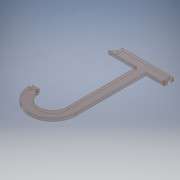
# Autodesk Inventor part: Liu_Inital_J
Saved by Autodesk Inventor 2017 (Build 210142000, 142)
## iProperties
Created: 2016-09-21
Part Number: Liu_Inital_J
Material: Polycarbonate, Smoke
Document SubType Name: Modeling
Designer: jliu
Density: 1.2 g/cm^3
Appearance: Polycarbonate - Smoked
Mass: 7.34155 g
Surface Area: 52.246 cm^2
Volume: 6.11796 cm^3
Author: jliu
Autodesk Inventor part; units mm, degrees
ref_plane "YZ Plane" through (0, 0, 0) normal (1, 0, 0) x (0, 1, 0)
ref_plane "XZ Plane" through (0, 0, 0) normal (0, 1, 0) x (-1, 0, 0)
ref_plane "XY Plane" through (0, 0, 0) normal (0, 0, 1) x (1, 0, 0)
sketch "Sketch1" plane through (0, 0, 0) normal (0, 0, 1) x (1, 0, 0)
  line L0 (5, 37.5) -> (5, -36.707)
  line L1 (-0.001, -37.5) -> (-0.001, 47.5) construction
  line L2 (-5.0021, 37.5) -> (-5.0021, -36.707)
  arc A0 (-44.9937, -37.5) -> (5, -36.707) centre (-19.9969, -37.1035) ccw
  arc A1 (-34.9916, -37.5) -> (-5.0021, -36.707) centre (-19.9969, -37.1035) ccw
  line L3 (5, 37.5) -> (24.9895, 37.5)
  line L4 (-24.9916, 47.5) -> (24.9895, 47.5)
  line L5 (-41.9937, -37.5) -> (-43.4937, -34.9019)
  line L6 (-41.9937, -37.5) -> (-38.9937, -37.5) construction
  line L7 (-44.9937, -37.5) -> (-41.9937, -37.5)
  line L8 (-34.9916, -37.5) -> (-37.9916, -37.5)
  line L9 (-37.9916, -37.5) -> (-36.4916, -34.9019)
  line L10 (-37.9916, -37.5) -> (-34.9916, -37.5) construction
  line L11 (-43.4937, -34.9019) -> (-36.4916, -34.9019)
  line L12 (-34.9916, -37.5) -> (-34.9916, 37.5) construction
  line L13 (-34.9916, -37.5) -> (40.0084, -37.5) construction
  line L14 (-5.0021, 37.5) -> (5, 37.5) construction
  line L15 (-34.9916, 37.5) -> (-5.0021, 37.5)
  line L16 (-34.9916, 37.5) -> (-20.8495, 37.5) construction
  line L17 (-29.9916, 42.5) -> (-29.9916, 47.5)
  line L18 (-29.9916, 47.5) -> (-24.9916, 47.5)
  line L19 (-34.9916, 37.5) -> (-29.9916, 42.5)
  line L20 (24.9895, 44.5) -> (21.9895, 46.2321)
  line L21 (24.9895, 40.5) -> (21.9895, 38.7679)
  line L22 (21.9895, 46.2321) -> (21.9895, 38.7679)
  line L23 (24.9895, 44.5) -> (24.9895, 47.5)
  line L24 (24.9895, 40.5) -> (24.9895, 37.5)
  point P0 (0, 0)
  dimension "d5" = 5
  dimension "d7" = 50
  dimension "d8" = 25
  dimension "d9" = 15
  dimension "d10" = 15
  dimension "d16" = 37.5
  dimension "d17" = 10
  dimension "d18" = 75
  dimension "d20" = 3
  dimension "d22" = 3
  dimension "d25" = 60
  dimension "d26" = 60
  dimension "d28" = 75
  dimension "d29" = 90
  dimension "d31" = 10
  dimension "d32" = 45
  dimension "d33" = 5
  dimension "d39" = 3
  dimension "d41" = 3
  dimension "d42" = 60
  dimension "d43" = 60
  dimension "d45" = 3
  dimension "d46" = 19.9895
  dimension "d47" = 24.9906
  dimension "d48" = 45.839
  constraints: 50 end point, 9 horizontal, 5 equal length, 4 point on circle, 3 collinear, 3 parallel, 3 symmetric about line, 3 vertical, 2 centre point, 1 coincident, 1 point on line
  measures "d5" distance from line of L0 point (0, 0)
  measures "d7" distance of L0.end L7.start
  measures "d8" radius of A0
  measures "d9" distance of L2.end A0.centre
  measures "d10" distance of L8.start A0.centre
  measures "d16" distance from line of point (0, 0) L3
  measures "d17" distance from line of L1.end L3
  measures "d18" distance from line of L1.start L3
  measures "d20" distance of L5.start L5.end
  measures "d22" distance of L7.start L5.start
  measures "d25" angle of L10 L9
  measures "d26" angle of L5 L7
  measures "d28" distance of L10.end L12.end
  measures "d29" angle of L13 L12
  measures "d31" distance of L3.end L4.end
  measures "d32" angle of L19 L15
  measures "d33" distance from line of L16 L17.start
  measures "d39" distance of L4.end L20.start
  measures "d41" distance of L3.end L21.start
  measures "d42" angle of L23 L20
  measures "d43" angle of L24 L21
  measures "d45" distance between parallel lines of L23 L22
  measures "d46" distance between parallel lines of L23 L0
  measures "d47" distance between parallel lines of L23 L1
  measures "d48" distance from line of L16.end L23
extrude "Extrusion1" add sketch "Sketch1" along normal blind 3.17
body "Solid1"
